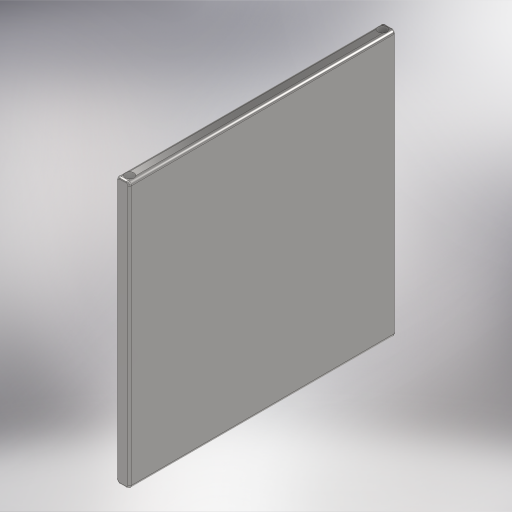
# Autodesk Inventor part: cata Beam
Saved by Autodesk Inventor 2024 (Build 280153000, 153)
## iProperties
Created: 2023-10-21
Part Number: cata Beam
Material: Stainless Steel
Document SubType Name: Modeling
Designer: aaron
Density: 8 g/cm^3
Appearance: Semi-Polished
Author: aaron
Autodesk Inventor part; units mm, degrees
ref_plane "YZ Plane" through (0, 0, 0) normal (1, 0, 0) x (0, 1, 0)
ref_plane "XZ Plane" through (0, 0, 0) normal (0, 1, 0) x (-1, 0, 0)
ref_plane "XY Plane" through (0, 0, 0) normal (0, 0, 1) x (1, 0, 0)
sketch "Sketch1" plane through (0, 0, 0) normal (0, 1, 0) x (-1, 0, 0)
  line L0 (3.175, -63.5) -> (-3.175, -63.5)
  line L1 (-3.175, -63.5) -> (-3.175, 63.5)
  line L2 (-3.175, 63.5) -> (3.175, 63.5)
  line L3 (3.175, 63.5) -> (3.175, -63.5)
  line L4 (3.175, -63.5) -> (-3.175, 63.5) construction
  line L5 (-3.175, -63.5) -> (3.175, 63.5) construction
  circle A0 centre (0, 60.325) radius 2.1082
  circle A1 centre (0, -60.325) radius 2.1082
  point P0 (0, 0)
  dimension "d0" = 6.35
  dimension "d1" = 127
  dimension "d2" = 4.2164
  dimension "d3" = 4.2164
  dimension "d4" = 3.175
  dimension "d5" = 3.175
  dimension "d6" = 3.175
  dimension "d7" = 3.175
  constraints: 12 end point, 2 centre point, 2 midpoint, 2 parallel, 1 horizontal, 1 perpendicular
  measures "d0" distance between parallel lines of L1 L3
  measures "d1" distance between parallel lines of L0 L2
  measures "d2" diameter of A1
  measures "d3" diameter of A0
  measures "d4" distance from line of L2 A0.centre
  measures "d5" distance from line of L0 A1.centre
  measures "d6" distance from line of L1 A0.centre
  measures "d7" distance from line of L1 A1.centre
extrude "Extrusion1" add sketch "Sketch1" along normal blind 127
fillet "Fillet1" radius 1.5875 4 edges at (3.175, 0, 0) (-3.175, 0, 0) (3.175, 127, 0) (-3.175, 127, 0)
fillet "Fillet2" radius 0.7937 16 edges at (0, 127, -63.5) (-2.71, 126.535, -63.5) (-3.175, 63.5, -63.5) (-2.71, 0.465, -63.5) (0, 0, -63.5) (2.71, 0.465, -63.5) (3.175, 63.5, -63.5) (2.71, 126.535, -63.5) (2.71, 126.535, 63.5) (0, 127, 63.5) (-2.71, 126.535, 63.5) (-3.175, 63.5, 63.5) (-2.71, 0.465, 63.5) (0, 0, 63.5) (2.71, 0.465, 63.5) (3.175, 63.5, 63.5)
equation "\"d8\" = d1"
body "Solid1"
